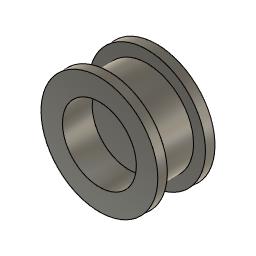
Side Wheel v6 (Autodesk Fusion 360 design; units mm, degrees)
Autodesk Fusion 360 part; units mm, degrees
note: some values were not read from the file. Set by a fixed rule: which sketch regions a step uses.
sketch "Sketch1" plane through (0, 0, 0) normal (1, 0, 0) x (0, 1, 0)
  line L0 (2.5, 0) -> (4.8, 0)
  line L1 (0, 4.9) -> (0.8, 4.9)
  line L2 (0.8, 4.9) -> (0.8, 3.9)
  line L3 (0.8, 3.9) -> (4, 3.9)
  line L4 (4, 3.9) -> (4, 4.9)
  line L5 (4, 4.9) -> (4.8, 4.9)
  line L6 (4.8, 4.9) -> (4.8, 0)
  line L7 (2.5, 0) -> (2.5, 3.1)
  line L8 (2.5, 3.1) -> (0, 3.1)
  line L9 (0, 3.1) -> (0, 4.9)
  dimension "d20" = 0.8
  dimension "d23" = 3.2
  dimension "d24" = 1
  dimension "d25" = 0.8
  dimension "d28" = 3.1
  constraint perpendicular L1 L2
  constraint perpendicular L3 L4
  constraint perpendicular L4 L5
  constraint perpendicular L0 L6
  constraint perpendicular L0 L7
  constraint perpendicular L7 L8
  constraint perpendicular L1 L9
  measures "d20" distance of L1.start L1.end
  measures "d23" distance of L2.end L3.end
  measures "d24" distance of L3.end L4.end
  measures "d25" distance of L4.end L5.end
  measures "d28" distance of L0.start L7.end
revolve "Revolve1" add sketch "Sketch1" angle 360 about axis through (0, 1.75, 0) along (0, 1, 0)
